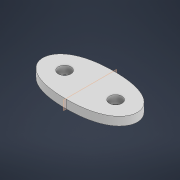
# Autodesk Inventor part: holder3_l1
Saved by Autodesk Inventor 2021 (Build 250183000, 183)
## iProperties
Created: 2021-06-13
Part Number: holder3_l1
Material: Generic
Document SubType Name: Modeling
Designer: Watchdog
Density: 1 g/cm^3
Appearance: Default
Author: Watchdog
Autodesk Inventor part; units mm, degrees
ref_plane "XZ Plane" through (0, 0, 0) normal (0, 1, 0) x (-1, 0, 0)
ref_plane "XY Plane" through (0, 0, 0) normal (0, 0, 1) x (1, 0, 0)
sketch "Sketch1" plane through (0, 0, 0) normal (0, 1, 0) x (-1, 0, 0)
  line L0 (0, 11.4356) -> (-24.4849, 11.4356) construction
  line L1 (-24.4849, 11.4356) -> (-27.1886, 0) construction
  line L2 (-27.1886, 0) -> (-24.4849, -11.325) construction
  line L3 (-24.4849, -11.325) -> (0, -11.325) construction
  spline S0 degree 4 poles (0, 11.4356) (-24.4849, 11.4356) (-27.1886, 0) (-24.4849, -11.325) (0, -11.325) knots 1 1 1 1 1 2 2 2 2 2
  line L4 (0, -122.0038) -> (0, 101.9612)
  line L5 (0, 11.4356) -> (24.4849, 11.4356) construction
  line L6 (24.4849, 11.4356) -> (27.1886, 0) construction
  line L7 (27.1886, 0) -> (24.4849, -11.325) construction
  line L8 (24.4849, -11.325) -> (0, -11.325) construction
  spline S1 degree 4 poles (0, 11.4356) (24.4849, 11.4356) (27.1886, 0) (24.4849, -11.325) (0, -11.325) knots 1 1 1 1 1 2 2 2 2 2
  point P0 (0, 0)
  constraints: 3 symmetric about line, 2 end point, 2 horizontal, 2 point on line, 1 vertical, 6 other
extrude "Extrusion1" add sketch "Sketch1" along normal blind 4
sketch "Sketch2" plane through (0, 4, 0) normal (0, 1, 0) x (1, 0, 0)
  point P0 (0, 0)
  point P1 (12.113, 0)
  point P2 (-12.113, 0)
  dimension "d2" = 12.113
  dimension "d10" = 12.113
  dimension "d11" = 0
  dimension "d12" = 0
  measures "d2" distance of point (0, 0) point (12.113, 0)
  measures "d10" distance of point (-12.113, 0) point (0, 0)
  measures "d11" vertical distance of point (0, 0) point (-12.113, 0)
  measures "d12" vertical distance of point (0, 0) point (12.113, 0)
hole "Hole1" at (12.113, 4, 0) at (-12.113, 4, 0) direction (0, -1, 0) diameter 6 end through all
equation "\"d10\" = d2"
body "Solid1"
